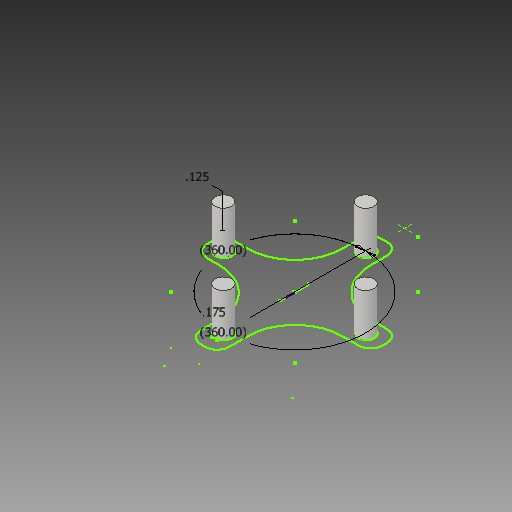
# Autodesk Inventor part: planetaryGearMt
Saved by Autodesk Inventor 2019 (Build 230136000, 136)
## iProperties
Created: 2019-10-26
Part Number: planetaryGearMt
Material: Generic
Document SubType Name: Modeling
Designer: test
Density: 1 g/cm^3
Appearance: Default
Author: test
Autodesk Inventor part; units mm, degrees
ref_plane "YZ Plane" through (0, 0, 0) normal (1, 0, 0) x (0, 1, 0)
ref_plane "XZ Plane" through (0, 0, 0) normal (0, 1, 0) x (-1, 0, 0)
sketch "Sketch1" plane through (0, 0, 0) normal (0, 1, 0) x (-1, 0, 0)
  circle A0 centre (0, 19.05) radius 2.2225
  circle A1 centre (-19.05, 0) radius 2.2225
  circle A2 centre (0, -19.05) radius 2.2225
  circle A3 centre (19.05, 0) radius 2.2225
  line L0 (0.635, 24.639) -> (-0.635, 24.639)
  line L1 (-0.635, -24.0273) -> (0.635, -24.0273)
  line L2 (0, 0) -> (0, 2.5439)
  line L3 (-24.0273, -0.635) -> (-24.0273, 0.635)
  line L4 (3.81, -20.8523) -> (3.81, -16.51)
  line L5 (3.81, 16.51) -> (3.81, 21.464)
  line L6 (-20.8523, 3.81) -> (-16.51, 3.81)
  line L7 (16.51, 3.81) -> (19.812, 3.81)
  line L8 (-3.81, 21.464) -> (-3.81, 16.51)
  line L9 (-3.81, -16.51) -> (-3.81, -20.8523)
  line L10 (19.812, -3.81) -> (16.51, -3.81)
  line L11 (-16.51, -3.81) -> (-20.8523, -3.81)
  arc A4 (3.81, 16.51) -> (16.51, 3.81) centre (16.51, 16.51) ccw
  arc A5 (16.51, -3.81) -> (3.81, -16.51) centre (16.51, -16.51) ccw
  arc A6 (-16.51, 3.81) -> (-3.81, 16.51) centre (-16.51, 16.51) ccw
  arc A7 (-3.81, -16.51) -> (-16.51, -3.81) centre (-16.51, -16.51) ccw
  line L12 (0, -3.81) -> (0, 0)
  line L13 (0, 3.81) -> (0, 0)
  line L14 (3.81, -20.8523) -> (3.81, -16.51)
  line L15 (16.51, 3.81) -> (19.812, 3.81)
  line L16 (21.2725, 0) -> (16.8275, 0)
  line L17 (19.812, 3.81) -> (16.51, 3.81)
  line L18 (19.812, -3.81) -> (16.51, -3.81)
  line L19 (0, -3.81) -> (0.635, -3.81)
  line L20 (16.51, -3.81) -> (19.812, -3.81)
  line L21 (-20.8523, -3.81) -> (-16.51, -3.81)
  line L22 (-3.81, -16.51) -> (-3.81, -20.8523)
  line L23 (0.635, -24.0273) -> (-0.635, -24.0273)
  line L24 (-3.81, -20.8523) -> (-3.81, -16.51)
  line L25 (0, 0) -> (0.635, 0)
  line L26 (-24.0273, 0.635) -> (-24.0273, -0.635)
  line L27 (-0.635, 24.639) -> (0.635, 24.639)
  line L28 (0.635, 0) -> (0, 0)
  line L29 (-3.81, 16.51) -> (-3.81, 21.464)
  line L30 (22.987, -0.635) -> (22.987, 0.635)
  arc A8 (0.635, 34.5382) -> (0, 34.544) centre (0, 0) ccw
  arc A9 (-24.0273, 24.8189) -> (-24.2117, 24.639) centre (0, 0) ccw
  line L31 (-20.8523, 3.81) -> (-16.51, 3.81)
  line L32 (-3.81, 29.464) -> (-3.81, 29.2166)
  line L33 (-3.81, 21.464) -> (-3.81, 16.51)
  line L34 (3.81, 29.464) -> (3.81, 29.2166)
  line L35 (3.81, 21.464) -> (3.81, 16.51)
  line L36 (3.81, 21.464) -> (3.81, 16.51)
  line L37 (19.812, 3.81) -> (16.51, 3.81)
  line L38 (16.51, -3.81) -> (19.812, -3.81)
  line L39 (3.81, -16.51) -> (3.81, -20.8523)
  line L40 (-20.8523, -3.81) -> (-16.51, -3.81)
  line L41 (0, -3.81) -> (0.635, -3.81)
  line L42 (0.635, 3.81) -> (0, 3.81)
  line L43 (-16.51, 3.81) -> (-20.8523, 3.81)
  arc A10 (19.812, -3.81) -> (22.987, -0.635) centre (19.812, -0.635) ccw
  arc A11 (22.987, 0.635) -> (19.812, 3.81) centre (19.812, 0.635) ccw
  arc A12 (3.81, 21.464) -> (0.635, 24.639) centre (0.635, 21.464) ccw
  arc A13 (-0.635, 24.639) -> (-3.81, 21.464) centre (-0.635, 21.464) ccw
  arc A14 (-20.8523, 3.81) -> (-24.0273, 0.635) centre (-20.8523, 0.635) ccw
  arc A15 (-24.0273, -0.635) -> (-20.8523, -3.81) centre (-20.8523, -0.635) ccw
  arc A16 (0.635, -24.0273) -> (3.81, -20.8523) centre (0.635, -20.8523) ccw
  arc A17 (-3.81, -20.8523) -> (-0.635, -24.0273) centre (-0.635, -20.8523) ccw
  point P0 (19.05, 0)
  point P1 (0, -19.05)
  point P2 (0, -29.464)
  point P3 (-3.81, -29.2166)
  dimension "d3" = 360
  dimension "d5" = 4.445
  dimension "d8" = 360
  dimension "d29" = 3.175
  constraints: 88 end point, 30 point on circle, 24 tangent, 18 centre point, 17 parallel, 10 equal radius, 8 horizontal, 5 perpendicular, 5 point on line, 1 coincident, 1 vertical, 14 other
  measures "d5" diameter of A0
  measures "d29" radius of A10
extrude "Extrusion4" add sketch "Sketch1" along normal blind 11.43 contours A0 | A1 | A2 | L16 A3 | A3 L16
ref_plane "Work Plane2" through (0, 5.08, 0) normal (0, 1, 0) x (1, 0, 0)
sketch "Sketch2" plane through (0, 5.08, 0) normal (0, 1, 0) x (1, 0, 0)
  circle A0 centre (0, 0) radius 2.8575
  dimension "d26" = 5.715
  constraints: 1 centre point, 1 coincident
  measures "d26" diameter of A0
extrude "Extrusion5" cut sketch "Sketch2" against normal blind 11.43
extrude "Extrusion6" cut sketch "Sketch1" along normal blind 5.08
extrude "Extrusion7" cut sketch "Sketch1" along normal blind 5.08
body "Solid2"
